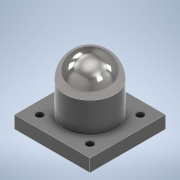
# Autodesk Inventor part: ballcaster
Saved by Autodesk Inventor 2022 (Build 260153000, 153)
## iProperties
Created: 2021-07-05
Part Number: ballcaster
Material: ポリプロピレン
Document SubType Name: Modeling
Designer: ken
Density: 0.899 g/cm^3
Appearance: 滑らか - 黒
Author: ken
Autodesk Inventor part; units mm, degrees
ref_plane "YZ Plane" through (0, 0, 0) normal (1, 0, 0) x (0, 1, 0)
ref_plane "XZ Plane" through (0, 0, 0) normal (0, 1, 0) x (-1, 0, 0)
ref_plane "XY Plane" through (0, 0, 0) normal (0, 0, 1) x (1, 0, 0)
sketch "スケッチ1" plane through (0, 0, 0) normal (0, 1, 0) x (-1, 0, 0)
  line L0 (0, 0) -> (30, 0)
  line L1 (30, 0) -> (30, -30)
  line L2 (30, -30) -> (0, -30)
  line L3 (0, -30) -> (0, 0)
  circle A0 centre (25, -5) radius 1.5
  circle A1 centre (25, -25) radius 1.5
  circle A2 centre (5, -5) radius 1.5
  circle A3 centre (5, -25) radius 1.5
  dimension "d18" = 30
  dimension "d19" = 30
  dimension "d20" = 3
  dimension "d21" = 3
  dimension "d22" = 20
  dimension "d23" = 5
  dimension "d24" = 5
  dimension "d25" = 3
  dimension "d26" = 3
  dimension "d27" = 20
  constraints: 8 end point, 4 centre point, 2 horizontal alignment, 2 parallel, 2 vertical alignment, 1 horizontal, 1 perpendicular
  measures "d18" distance of L1.end L2.end
  measures "d19" distance of L0.end L1.end
  measures "d20" diameter of A0
  measures "d21" diameter of A1
  measures "d22" distance of A0.centre A1.centre
  measures "d23" distance from line of L2 A1.centre
  measures "d24" distance from line of L1 A1.centre
  measures "d25" diameter of A2
  measures "d26" diameter of A3
  measures "d27" distance of A3.centre A1.centre
extrude "押し出し1" add sketch "スケッチ1" along normal blind 5
sketch "スケッチ2" plane through (0, 5, 0) normal (0, 1, 0) x (1, 0, 0)
  circle A0 centre (-15, 15) radius 10
  line L0 (0, 30) -> (-30, 30) projected
  line L1 (-30, 30) -> (-30, 0) projected
  point P0 (0, 0)
  dimension "d32" = 20
  dimension "d33" = 15
  dimension "d34" = 15
  constraints: 1 centre point
  measures "d32" diameter of A0
  measures "d33" distance from line of L0 A0.centre
  measures "d34" distance from line of A0.centre L1
extrude "押し出し2" add sketch "スケッチ2" along normal blind 12
sketch "スケッチ9" plane through (-15, 17, -15) normal (0, 1, 0) x (1, 0, 0)
  circle A0 centre (0, 0) radius 10 projected
  circle A1 centre (0, 0) radius 10 projected
  point P0 (15, -15)
extrude "押し出し4" add sketch "スケッチ9" along normal blind 10
fillet "フィレット1" radius 10 1 edges at (-25, 27, -15)
